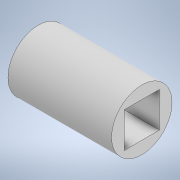
# Autodesk Inventor part: 220411 Small Rod Plain
Saved by Autodesk Inventor 2022 (Build 260153000, 153)
## iProperties
Created: 2022-01-27
Part Number: 220411 Small Rod Plain
Material: Generic
Document SubType Name: Modeling
Designer: josephinew
Density: 1 g/cm^3
Appearance: Default
Author: josephinew
Autodesk Inventor part; units mm, degrees
ref_plane "YZ Plane" through (0, 0, 0) normal (1, 0, 0) x (0, 1, 0)
ref_plane "XZ Plane" through (0, 0, 0) normal (0, 1, 0) x (-1, 0, 0)
ref_plane "XY Plane" through (0, 0, 0) normal (0, 0, 1) x (1, 0, 0)
sketch "Sketch1" plane through (0, 0, 0) normal (1, 0, 0) x (0, 1, 0)
  circle A0 centre (0, 0) radius 22.225
  line L0 (12.954, 12.954) -> (-12.954, 12.954)
  line L1 (-12.954, 12.954) -> (-12.954, -12.954)
  line L2 (-12.954, -12.954) -> (12.954, -12.954)
  line L3 (12.954, -12.954) -> (12.954, 12.954)
  dimension "d0" = 44.45
  dimension "d1" = 25.908
  dimension "d2" = 25.908
  constraints: 8 end point, 2 parallel, 1 centre point, 1 coincident, 1 horizontal, 1 perpendicular
  measures "d0" diameter of A0
  measures "d1" distance of L2.end L1.end
  measures "d2" distance of L1.end L0.end
extrude "Extrusion1" add sketch "Sketch1" along normal blind 76.2
body "Solid1"
